Autodesk Fusion 360 part; units mm, degrees
(part 2 of 14)
sketch "Sketch8" plane through (0, 0, 5) normal (0, 0, 1) x (-1, 0, 0)
  spline S0 degree 5 poles (-28.167, 1.1579) (-28.1751, 1.1579) (-28.1914, 1.1578) (-28.2159, 1.1575) (-28.2485, 1.1567) (-28.2892, 1.1551) (-28.33, 1.1529) (-28.3707, 1.1501) (-28.4115, 1.1467) (-28.4523, 1.1427) (-28.493, 1.1383) (-28.5338, 1.1335) (-28.5746, 1.1284) (-28.6154, 1.1228) (-28.6561, 1.117) (-28.6969, 1.1109) (-28.7376, 1.1045) (-28.7783, 1.0977) (-28.8191, 1.0907) (-28.8598, 1.0834) (-28.9005, 1.0758) (-28.9412, 1.0679) (-28.9819, 1.0597) (-29.0226, 1.0513) (-29.0633, 1.0427) (-29.104, 1.0338) (-29.1446, 1.0247) (-29.1853, 1.0153) (-29.2259, 1.0057) (-29.2665, 0.9959) (-29.3071, 0.9858) (-29.3477, 0.9755) (-29.3883, 0.965) (-29.4289, 0.9543) (-29.4694, 0.9434) (-29.5099, 0.9323) (-29.5505, 0.921) (-29.591, 0.9094) (-29.6315, 0.8977) (-29.672, 0.8858) (-29.7124, 0.8737) (-29.7529, 0.8614) (-29.7933, 0.8488) (-29.8337, 0.8361) (-29.8741, 0.8233) (-29.9145, 0.8102) (-29.9549, 0.7969) (-29.9952, 0.7835) (-30.0355, 0.7699) (-30.0759, 0.7561) (-30.1161, 0.7421) (-30.1564, 0.728) (-30.1967, 0.7137) (-30.2369, 0.6992) (-30.2771, 0.6845) (-30.3173, 0.6697) (-30.3575, 0.6547) (-30.3977, 0.6396) (-30.4378, 0.6242) (-30.4779, 0.6087) (-30.518, 0.5931) (-30.5581, 0.5773) (-30.5982, 0.5613) (-30.6382, 0.5451) (-30.6782, 0.5288) (-30.7182, 0.5124) (-30.7582, 0.4958) (-30.7981, 0.479) (-30.838, 0.4621) (-30.8779, 0.445) (-30.9178, 0.4278) (-30.9497, 0.4139) (-30.9736, 0.4034) (-30.9895, 0.3963) (-30.9975, 0.3928) knots 0 0 0 0 0 0 0.01428571 0.02857143 0.04285714 0.05714286 0.07142857 0.08571429 0.1 0.11428571 0.12857143 0.14285714 0.15714286 0.17142857 0.18571429 0.2 0.21428571 0.22857143 0.24285714 0.25714286 0.27142857 0.28571429 0.3 0.31428571 0.32857143 0.34285714 0.35714286 0.37142857 0.38571429 0.4 0.41428571 0.42857143 0.44285714 0.45714286 0.47142857 0.48571429 0.5 0.51428571 0.52857143 0.54285714 0.55714286 0.57142857 0.58571429 0.6 0.61428571 0.62857143 0.64285714 0.65714286 0.67142857 0.68571429 0.7 0.71428571 0.72857143 0.74285714 0.75714286 0.77142857 0.78571429 0.8 0.81428571 0.82857143 0.84285714 0.85714286 0.87142857 0.88571429 0.9 0.91428571 0.92857143 0.94285714 0.95714286 0.97142857 0.98571429 1 1 1 1 1 1
  arc A0 (-30.9975, 0.3928) -> (-30.9975, -0.3928) centre (0, 0) ccw
  spline S1 degree 5 poles (-30.9975, -0.3928) (-30.9895, -0.3963) (-30.9736, -0.4034) (-30.9497, -0.4139) (-30.9178, -0.4278) (-30.8779, -0.445) (-30.838, -0.4621) (-30.7981, -0.479) (-30.7582, -0.4958) (-30.7182, -0.5124) (-30.6782, -0.5288) (-30.6382, -0.5451) (-30.5982, -0.5613) (-30.5581, -0.5773) (-30.518, -0.5931) (-30.4779, -0.6087) (-30.4378, -0.6242) (-30.3977, -0.6396) (-30.3575, -0.6547) (-30.3173, -0.6697) (-30.2771, -0.6845) (-30.2369, -0.6992) (-30.1967, -0.7137) (-30.1564, -0.728) (-30.1161, -0.7421) (-30.0759, -0.7561) (-30.0355, -0.7699) (-29.9952, -0.7835) (-29.9549, -0.7969) (-29.9145, -0.8102) (-29.8741, -0.8233) (-29.8337, -0.8361) (-29.7933, -0.8488) (-29.7529, -0.8614) (-29.7124, -0.8737) (-29.672, -0.8858) (-29.6315, -0.8977) (-29.591, -0.9094) (-29.5505, -0.921) (-29.5099, -0.9323) (-29.4694, -0.9434) (-29.4289, -0.9543) (-29.3883, -0.965) (-29.3477, -0.9755) (-29.3071, -0.9858) (-29.2665, -0.9959) (-29.2259, -1.0057) (-29.1853, -1.0153) (-29.1446, -1.0247) (-29.104, -1.0338) (-29.0633, -1.0427) (-29.0226, -1.0513) (-28.9819, -1.0597) (-28.9412, -1.0679) (-28.9005, -1.0758) (-28.8598, -1.0834) (-28.8191, -1.0907) (-28.7783, -1.0977) (-28.7376, -1.1045) (-28.6969, -1.1109) (-28.6561, -1.117) (-28.6154, -1.1228) (-28.5746, -1.1284) (-28.5338, -1.1335) (-28.493, -1.1383) (-28.4523, -1.1427) (-28.4115, -1.1467) (-28.3707, -1.1501) (-28.33, -1.1529) (-28.2892, -1.1551) (-28.2485, -1.1567) (-28.2159, -1.1575) (-28.1914, -1.1578) (-28.1751, -1.1579) (-28.167, -1.1579) knots -1 -1 -1 -1 -1 -1 -0.98571429 -0.97142857 -0.95714286 -0.94285714 -0.92857143 -0.91428571 -0.9 -0.88571429 -0.87142857 -0.85714286 -0.84285714 -0.82857143 -0.81428571 -0.8 -0.78571429 -0.77142857 -0.75714286 -0.74285714 -0.72857143 -0.71428571 -0.7 -0.68571429 -0.67142857 -0.65714286 -0.64285714 -0.62857143 -0.61428571 -0.6 -0.58571429 -0.57142857 -0.55714286 -0.54285714 -0.52857143 -0.51428571 -0.5 -0.48571429 -0.47142857 -0.45714286 -0.44285714 -0.42857143 -0.41428571 -0.4 -0.38571429 -0.37142857 -0.35714286 -0.34285714 -0.32857143 -0.31428571 -0.3 -0.28571429 -0.27142857 -0.25714286 -0.24285714 -0.22857143 -0.21428571 -0.2 -0.18571429 -0.17142857 -0.15714286 -0.14285714 -0.12857143 -0.11428571 -0.1 -0.08571429 -0.07142857 -0.05714286 -0.04285714 -0.02857143 -0.01428571 0 0 0 0 0 0
  spline S2 degree 5 poles (-28.1337, -1.7927) (-28.1418, -1.7936) (-28.158, -1.7954) (-28.1823, -1.7982) (-28.2146, -1.8024) (-28.255, -1.8083) (-28.2953, -1.8147) (-28.3355, -1.8218) (-28.3757, -1.8294) (-28.4159, -1.8376) (-28.4559, -1.8462) (-28.496, -1.8553) (-28.536, -1.8647) (-28.576, -1.8744) (-28.6159, -1.8845) (-28.6558, -1.8948) (-28.6956, -1.9055) (-28.7354, -1.9164) (-28.7752, -1.9277) (-28.815, -1.9392) (-28.8546, -1.9511) (-28.8943, -1.9632) (-28.9339, -1.9755) (-28.9735, -1.9881) (-29.0131, -2.001) (-29.0526, -2.0141) (-29.0921, -2.0274) (-29.1315, -2.041) (-29.1709, -2.0548) (-29.2103, -2.0688) (-29.2496, -2.083) (-29.2889, -2.0975) (-29.3282, -2.1122) (-29.3674, -2.127) (-29.4066, -2.1421) (-29.4457, -2.1574) (-29.4849, -2.1729) (-29.5239, -2.1886) (-29.563, -2.2045) (-29.602, -2.2206) (-29.641, -2.2369) (-29.6799, -2.2534) (-29.7188, -2.2701) (-29.7577, -2.2869) (-29.7965, -2.3039) (-29.8353, -2.3212) (-29.8741, -2.3386) (-29.9128, -2.3561) (-29.9515, -2.3739) (-29.9901, -2.3918) (-30.0287, -2.4099) (-30.0673, -2.4282) (-30.1059, -2.4466) (-30.1444, -2.4653) (-30.1828, -2.484) (-30.2213, -2.503) (-30.2596, -2.5221) (-30.298, -2.5414) (-30.3363, -2.5608) (-30.3746, -2.5804) (-30.4128, -2.6002) (-30.451, -2.6201) (-30.4892, -2.6402) (-30.5273, -2.6604) (-30.5654, -2.6808) (-30.6035, -2.7013) (-30.6415, -2.722) (-30.6795, -2.7429) (-30.7174, -2.7639) (-30.7553, -2.7851) (-30.7932, -2.8064) (-30.8234, -2.8235) (-30.8461, -2.8365) (-30.8612, -2.8451) (-30.8688, -2.8495) knots 0 0 0 0 0 0 0.01428571 0.02857143 0.04285714 0.05714286 0.07142857 0.08571429 0.1 0.11428571 0.12857143 0.14285714 0.15714286 0.17142857 0.18571429 0.2 0.21428571 0.22857143 0.24285714 0.25714286 0.27142857 0.28571429 0.3 0.31428571 0.32857143 0.34285714 0.35714286 0.37142857 0.38571429 0.4 0.41428571 0.42857143 0.44285714 0.45714286 0.47142857 0.48571429 0.5 0.51428571 0.52857143 0.54285714 0.55714286 0.57142857 0.58571429 0.6 0.61428571 0.62857143 0.64285714 0.65714286 0.67142857 0.68571429 0.7 0.71428571 0.72857143 0.74285714 0.75714286 0.77142857 0.78571429 0.8 0.81428571 0.82857143 0.84285714 0.85714286 0.87142857 0.88571429 0.9 0.91428571 0.92857143 0.94285714 0.95714286 0.97142857 0.98571429 1 1 1 1 1 1
  arc A1 (-30.8688, -2.8495) -> (-30.7866, -3.6308) centre (0, 0) ccw
  spline S3 degree 5 poles (-30.7866, -3.6308) (-30.7784, -3.6335) (-30.7618, -3.6388) (-30.7369, -3.6467) (-30.7037, -3.6572) (-30.6623, -3.6702) (-30.6208, -3.683) (-30.5793, -3.6957) (-30.5379, -3.7082) (-30.4964, -3.7205) (-30.4549, -3.7327) (-30.4134, -3.7447) (-30.3719, -3.7566) (-30.3304, -3.7683) (-30.2889, -3.7798) (-30.2473, -3.7912) (-30.2058, -3.8024) (-30.1643, -3.8135) (-30.1228, -3.8244) (-30.0812, -3.8351) (-30.0397, -3.8456) (-29.9982, -3.856) (-29.9567, -3.8662) (-29.9151, -3.8762) (-29.8736, -3.8861) (-29.8321, -3.8958) (-29.7905, -3.9053) (-29.749, -3.9146) (-29.7075, -3.9237) (-29.6659, -3.9327) (-29.6244, -3.9415) (-29.5829, -3.95) (-29.5414, -3.9584) (-29.4998, -3.9667) (-29.4583, -3.9747) (-29.4168, -3.9825) (-29.3753, -3.9901) (-29.3338, -3.9976) (-29.2923, -4.0048) (-29.2508, -4.0118) (-29.2094, -4.0186) (-29.1679, -4.0253) (-29.1264, -4.0317) (-29.085, -4.0379) (-29.0435, -4.0438) (-29.0021, -4.0496) (-28.9607, -4.0551) (-28.9192, -4.0604) (-28.8778, -4.0655) (-28.8365, -4.0703) (-28.7951, -4.0749) (-28.7537, -4.0792) (-28.7124, -4.0833) (-28.6711, -4.0872) (-28.6298, -4.0908) (-28.5885, -4.0941) (-28.5472, -4.0971) (-28.506, -4.0999) (-28.4647, -4.1023) (-28.4235, -4.1044) (-28.3824, -4.1063) (-28.3412, -4.1078) (-28.3001, -4.109) (-28.259, -4.1099) (-28.218, -4.1104) (-28.177, -4.1106) (-28.136, -4.1102) (-28.0951, -4.1093) (-28.0543, -4.1078) (-28.0135, -4.1058) (-27.9728, -4.1031) (-27.9403, -4.1005) (-27.916, -4.0983) (-27.8998, -4.0966) (-27.8917, -4.0958) knots -1 -1 -1 -1 -1 -1 -0.98571429 -0.97142857 -0.95714286 -0.94285714 -0.92857143 -0.91428571 -0.9 -0.88571429 -0.87142857 -0.85714286 -0.84285714 -0.82857143 -0.81428571 -0.8 -0.78571429 -0.77142857 -0.75714286 -0.74285714 -0.72857143 -0.71428571 -0.7 -0.68571429 -0.67142857 -0.65714286 -0.64285714 -0.62857143 -0.61428571 -0.6 -0.58571429 -0.57142857 -0.55714286 -0.54285714 -0.52857143 -0.51428571 -0.5 -0.48571429 -0.47142857 -0.45714286 -0.44285714 -0.42857143 -0.41428571 -0.4 -0.38571429 -0.37142857 -0.35714286 -0.34285714 -0.32857143 -0.31428571 -0.3 -0.28571429 -0.27142857 -0.25714286 -0.24285714 -0.22857143 -0.21428571 -0.2 -0.18571429 -0.17142857 -0.15714286 -0.14285714 -0.12857143 -0.11428571 -0.1 -0.08571429 -0.07142857 -0.05714286 -0.04285714 -0.02857143 -0.01428571 0 0 0 0 0 0
  spline S4 degree 5 poles (-27.7922, -4.7237) (-27.8002, -4.7254) (-27.8161, -4.7288) (-27.8399, -4.7342) (-27.8717, -4.7418) (-27.9112, -4.7518) (-27.9506, -4.7625) (-27.9899, -4.7737) (-28.029, -4.7855) (-28.0681, -4.7978) (-28.1071, -4.8106) (-28.146, -4.8237) (-28.1848, -4.8373) (-28.2235, -4.8512) (-28.2621, -4.8653) (-28.3007, -4.8798) (-28.3393, -4.8946) (-28.3777, -4.9096) (-28.4161, -4.925) (-28.4544, -4.9406) (-28.4926, -4.9565) (-28.5308, -4.9727) (-28.5689, -4.9891) (-28.607, -5.0058) (-28.645, -5.0227) (-28.6829, -5.0399) (-28.7208, -5.0572) (-28.7586, -5.0749) (-28.7963, -5.0927) (-28.834, -5.1107) (-28.8716, -5.129) (-28.9092, -5.1475) (-28.9467, -5.1662) (-28.9842, -5.1851) (-29.0216, -5.2042) (-29.0589, -5.2235) (-29.0962, -5.243) (-29.1334, -5.2627) (-29.1706, -5.2826) (-29.2077, -5.3027) (-29.2448, -5.323) (-29.2818, -5.3434) (-29.3187, -5.3641) (-29.3556, -5.3849) (-29.3925, -5.4059) (-29.4292, -5.4271) (-29.466, -5.4484) (-29.5026, -5.47) (-29.5393, -5.4917) (-29.5758, -5.5135) (-29.6123, -5.5356) (-29.6488, -5.5578) (-29.6852, -5.5802) (-29.7215, -5.6027) (-29.7578, -5.6254) (-29.7941, -5.6483) (-29.8303, -5.6713) (-29.8664, -5.6945) (-29.9025, -5.7178) (-29.9385, -5.7413) (-29.9744, -5.7649) (-30.0104, -5.7887) (-30.0462, -5.8127) (-30.082, -5.8368) (-30.1178, -5.8611) (-30.1535, -5.8855) (-30.1891, -5.91) (-30.2247, -5.9348) (-30.2602, -5.9596) (-30.2957, -5.9846) (-30.3311, -6.0097) (-30.3594, -6.03) (-30.3806, -6.0452) (-30.3948, -6.0554) (-30.4018, -6.0605) knots 0 0 0 0 0 0 0.01428571 0.02857143 0.04285714 0.05714286 0.07142857 0.08571429 0.1 0.11428571 0.12857143 0.14285714 0.15714286 0.17142857 0.18571429 0.2 0.21428571 0.22857143 0.24285714 0.25714286 0.27142857 0.28571429 0.3 0.31428571 0.32857143 0.34285714 0.35714286 0.37142857 0.38571429 0.4 0.41428571 0.42857143 0.44285714 0.45714286 0.47142857 0.48571429 0.5 0.51428571 0.52857143 0.54285714 0.55714286 0.57142857 0.58571429 0.6 0.61428571 0.62857143 0.64285714 0.65714286 0.67142857 0.68571429 0.7 0.71428571 0.72857143 0.74285714 0.75714286 0.77142857 0.78571429 0.8 0.81428571 0.82857143 0.84285714 0.85714286 0.87142857 0.88571429 0.9 0.91428571 0.92857143 0.94285714 0.95714286 0.97142857 0.98571429 1 1 1 1 1 1
  arc A2 (-30.4018, -6.0605) -> (-30.2385, -6.829) centre (0, 0) ccw
  spline S5 degree 5 poles (-30.2385, -6.829) (-30.2299, -6.8308) (-30.2129, -6.8343) (-30.1873, -6.8396) (-30.1533, -6.8466) (-30.1107, -6.8552) (-30.0681, -6.8636) (-30.0255, -6.8718) (-29.983, -6.8799) (-29.9404, -6.8879) (-29.8979, -6.8956) (-29.8553, -6.9033) (-29.8128, -6.9107) (-29.7703, -6.918) (-29.7278, -6.9252) (-29.6854, -6.9321) (-29.6429, -6.939) (-29.6004, -6.9456) (-29.558, -6.9521) (-29.5156, -6.9584) (-29.4732, -6.9646) (-29.4308, -6.9705) (-29.3884, -6.9763) (-29.3461, -6.982) (-29.3037, -6.9874) (-29.2614, -6.9927) (-29.2191, -6.9978) (-29.1768, -7.0027) (-29.1346, -7.0075) (-29.0923, -7.0121) (-29.0501, -7.0165) (-29.0079, -7.0207) (-28.9658, -7.0247) (-28.9236, -7.0285) (-28.8815, -7.0321) (-28.8394, -7.0356) (-28.7973, -7.0388) (-28.7553, -7.0419) (-28.7132, -7.0447) (-28.6712, -7.0474) (-28.6293, -7.0498) (-28.5873, -7.0521) (-28.5454, -7.0541) (-28.5036, -7.0559) (-28.4617, -7.0576) (-28.4199, -7.059) (-28.3781, -7.0601) (-28.3364, -7.0611) (-28.2947, -7.0618) (-28.253, -7.0622) (-28.2114, -7.0625) (-28.1698, -7.0625) (-28.1283, -7.0622) (-28.0868, -7.0618) (-28.0453, -7.061) (-28.0039, -7.06) (-27.9625, -7.0587) (-27.9212, -7.0571) (-27.88, -7.0552) (-27.8388, -7.053) (-27.7977, -7.0505) (-27.7566, -7.0478) (-27.7156, -7.0447) (-27.6746, -7.0413) (-27.6337, -7.0375) (-27.5929, -7.0333) (-27.5522, -7.0287) (-27.5117, -7.0235) (-27.4712, -7.0178) (-27.4309, -7.0115) (-27.3907, -7.0046) (-27.3586, -6.9986) (-27.3347, -6.9938) (-27.3187, -6.9905) (-27.3107, -6.9888) knots -1 -1 -1 -1 -1 -1 -0.98571429 -0.97142857 -0.95714286 -0.94285714 -0.92857143 -0.91428571 -0.9 -0.88571429 -0.87142857 -0.85714286 -0.84285714 -0.82857143 -0.81428571 -0.8 -0.78571429 -0.77142857 -0.75714286 -0.74285714 -0.72857143 -0.71428571 -0.7 -0.68571429 -0.67142857 -0.65714286 -0.64285714 -0.62857143 -0.61428571 -0.6 -0.58571429 -0.57142857 -0.55714286 -0.54285714 -0.52857143 -0.51428571 -0.5 -0.48571429 -0.47142857 -0.45714286 -0.44285714 -0.42857143 -0.41428571 -0.4 -0.38571429 -0.37142857 -0.35714286 -0.34285714 -0.32857143 -0.31428571 -0.3 -0.28571429 -0.27142857 -0.25714286 -0.24285714 -0.22857143 -0.21428571 -0.2 -0.18571429 -0.17142857 -0.15714286 -0.14285714 -0.12857143 -0.11428571 -0.1 -0.08571429 -0.07142857 -0.05714286 -0.04285714 -0.02857143 -0.01428571 0 0 0 0 0 0
  spline S6 degree 5 poles (-27.1462, -7.6029) (-27.1539, -7.6054) (-27.1694, -7.6105) (-27.1926, -7.6184) (-27.2233, -7.6292) (-27.2616, -7.6433) (-27.2997, -7.658) (-27.3376, -7.6733) (-27.3753, -7.6891) (-27.4128, -7.7054) (-27.4503, -7.7222) (-27.4876, -7.7394) (-27.5247, -7.7569) (-27.5618, -7.7747) (-27.5988, -7.7929) (-27.6356, -7.8113) (-27.6724, -7.83) (-27.7091, -7.849) (-27.7456, -7.8683) (-27.7821, -7.8878) (-27.8185, -7.9076) (-27.8547, -7.9277) (-27.8909, -7.9481) (-27.927, -7.9686) (-27.963, -7.9894) (-27.999, -8.0104) (-28.0348, -8.0317) (-28.0706, -8.0531) (-28.1062, -8.0748) (-28.1418, -8.0967) (-28.1774, -8.1188) (-28.2128, -8.1412) (-28.2481, -8.1637) (-28.2834, -8.1864) (-28.3186, -8.2093) (-28.3537, -8.2324) (-28.3888, -8.2557) (-28.4237, -8.2792) (-28.4586, -8.3028) (-28.4934, -8.3267) (-28.5282, -8.3507) (-28.5628, -8.3749) (-28.5974, -8.3993) (-28.6319, -8.4239) (-28.6664, -8.4486) (-28.7007, -8.4735) (-28.735, -8.4986) (-28.7693, -8.5239) (-28.8034, -8.5493) (-28.8375, -8.5748) (-28.8715, -8.6006) (-28.9054, -8.6265) (-28.9393, -8.6525) (-28.9731, -8.6787) (-29.0068, -8.7051) (-29.0405, -8.7316) (-29.074, -8.7583) (-29.1075, -8.7851) (-29.141, -8.8121) (-29.1743, -8.8393) (-29.2076, -8.8665) (-29.2409, -8.894) (-29.274, -8.9215) (-29.3071, -8.9493) (-29.3401, -8.9771) (-29.3731, -9.0051) (-29.406, -9.0333) (-29.4388, -9.0616) (-29.4715, -9.09) (-29.5042, -9.1186) (-29.5368, -9.1473) (-29.5628, -9.1704) (-29.5823, -9.1877) (-29.5953, -9.1994) (-29.6018, -9.2052) knots 0 0 0 0 0 0 0.01428571 0.02857143 0.04285714 0.05714286 0.07142857 0.08571429 0.1 0.11428571 0.12857143 0.14285714 0.15714286 0.17142857 0.18571429 0.2 0.21428571 0.22857143 0.24285714 0.25714286 0.27142857 0.28571429 0.3 0.31428571 0.32857143 0.34285714 0.35714286 0.37142857 0.38571429 0.4 0.41428571 0.42857143 0.44285714 0.45714286 0.47142857 0.48571429 0.5 0.51428571 0.52857143 0.54285714 0.55714286 0.57142857 0.58571429 0.6 0.61428571 0.62857143 0.64285714 0.65714286 0.67142857 0.68571429 0.7 0.71428571 0.72857143 0.74285714 0.75714286 0.77142857 0.78571429 0.8 0.81428571 0.82857143 0.84285714 0.85714286 0.87142857 0.88571429 0.9 0.91428571 0.92857143 0.94285714 0.95714286 0.97142857 0.98571429 1 1 1 1 1 1
  arc A3 (-29.6018, -9.2052) -> (-29.359, -9.9524) centre (0, 0) ccw
  spline S7 degree 5 poles (-29.359, -9.9524) (-29.3503, -9.9532) (-29.333, -9.955) (-29.307, -9.9576) (-29.2724, -9.961) (-29.2292, -9.965) (-29.1859, -9.9689) (-29.1427, -9.9727) (-29.0996, -9.9763) (-29.0564, -9.9798) (-29.0133, -9.983) (-28.9702, -9.9862) (-28.9271, -9.9892) (-28.8841, -9.992) (-28.8411, -9.9946) (-28.7981, -9.9971) (-28.7552, -9.9995) (-28.7123, -10.0016) (-28.6694, -10.0037) (-28.6265, -10.0055) (-28.5837, -10.0072) (-28.541, -10.0087) (-28.4982, -10.01) (-28.4555, -10.0112) (-28.4128, -10.0122) (-28.3702, -10.0131) (-28.3276, -10.0137) (-28.285, -10.0142) (-28.2425, -10.0145) (-28.2, -10.0146) (-28.1576, -10.0146) (-28.1152, -10.0144) (-28.0728, -10.0139) (-28.0305, -10.0133) (-27.9882, -10.0126) (-27.946, -10.0116) (-27.9038, -10.0104) (-27.8617, -10.0091) (-27.8196, -10.0075) (-27.7775, -10.0057) (-27.7355, -10.0038) (-27.6936, -10.0016) (-27.6517, -9.9993) (-27.6099, -9.9967) (-27.5681, -9.994) (-27.5264, -9.991) (-27.4847, -9.9878) (-27.4431, -9.9843) (-27.4015, -9.9807) (-27.3601, -9.9768) (-27.3186, -9.9727) (-27.2773, -9.9683) (-27.236, -9.9638) (-27.1948, -9.9589) (-27.1536, -9.9539) (-27.1125, -9.9485) (-27.0715, -9.9429) (-27.0306, -9.937) (-26.9898, -9.9308) (-26.9491, -9.9243) (-26.9084, -9.9176) (-26.8678, -9.9105) (-26.8274, -9.9032) (-26.787, -9.8955) (-26.7467, -9.8875) (-26.7066, -9.879) (-26.6666, -9.8702) (-26.6268, -9.8608) (-26.5871, -9.8509) (-26.5477, -9.8404) (-26.5084, -9.8293) (-26.4772, -9.82) (-26.4539, -9.8128) (-26.4383, -9.8078) (-26.4306, -9.8053) knots -1 -1 -1 -1 -1 -1 -0.98571429 -0.97142857 -0.95714286 -0.94285714 -0.92857143 -0.91428571 -0.9 -0.88571429 -0.87142857 -0.85714286 -0.84285714 -0.82857143 -0.81428571 -0.8 -0.78571429 -0.77142857 -0.75714286 -0.74285714 -0.72857143 -0.71428571 -0.7 -0.68571429 -0.67142857 -0.65714286 -0.64285714 -0.62857143 -0.61428571 -0.6 -0.58571429 -0.57142857 -0.55714286 -0.54285714 -0.52857143 -0.51428571 -0.5 -0.48571429 -0.47142857 -0.45714286 -0.44285714 -0.42857143 -0.41428571 -0.4 -0.38571429 -0.37142857 -0.35714286 -0.34285714 -0.32857143 -0.31428571 -0.3 -0.28571429 -0.27142857 -0.25714286 -0.24285714 -0.22857143 -0.21428571 -0.2 -0.18571429 -0.17142857 -0.15714286 -0.14285714 -0.12857143 -0.11428571 -0.1 -0.08571429 -0.07142857 -0.05714286 -0.04285714 -0.02857143 -0.01428571 0 0 0 0 0 0
  spline S8 degree 5 poles (-26.2028, -10.3988) (-26.2102, -10.4021) (-26.2251, -10.4088) (-26.2473, -10.419) (-26.2767, -10.433) (-26.3133, -10.451) (-26.3496, -10.4696) (-26.3857, -10.4888) (-26.4216, -10.5085) (-26.4572, -10.5286) (-26.4927, -10.5492) (-26.528, -10.5702) (-26.5631, -10.5915) (-26.5981, -10.6131) (-26.633, -10.635) (-26.6677, -10.6572) (-26.7023, -10.6797) (-26.7368, -10.7024) (-26.7712, -10.7254) (-26.8054, -10.7486) (-26.8395, -10.7721) (-26.8735, -10.7959) (-26.9073, -10.8199) (-26.9411, -10.8441) (-26.9747, -10.8686) (-27.0083, -10.8932) (-27.0417, -10.9181) (-27.075, -10.9432) (-27.1082, -10.9685) (-27.1413, -10.994) (-27.1743, -11.0197) (-27.2073, -11.0456) (-27.2401, -11.0717) (-27.2728, -11.098) (-27.3054, -11.1244) (-27.3379, -11.1511) (-27.3703, -11.1779) (-27.4026, -11.2049) (-27.4348, -11.2321) (-27.467, -11.2595) (-27.499, -11.287) (-27.5309, -11.3147) (-27.5628, -11.3426) (-27.5946, -11.3706) (-27.6262, -11.3988) (-27.6578, -11.4272) (-27.6893, -11.4557) (-27.7207, -11.4844) (-27.752, -11.5132) (-27.7832, -11.5422) (-27.8143, -11.5714) (-27.8454, -11.6007) (-27.8763, -11.6301) (-27.9072, -11.6597) (-27.938, -11.6895) (-27.9687, -11.7194) (-27.9993, -11.7494) (-28.0298, -11.7796) (-28.0602, -11.8099) (-28.0906, -11.8404) (-28.1208, -11.871) (-28.151, -11.9018) (-28.1811, -11.9326) (-28.2111, -11.9637) (-28.241, -11.9948) (-28.2709, -12.0261) (-28.3006, -12.0576) (-28.3303, -12.0891) (-28.3599, -12.1208) (-28.3894, -12.1527) (-28.4188, -12.1846) (-28.4423, -12.2103) (-28.4599, -12.2296) (-28.4716, -12.2425) (-28.4774, -12.249) knots 0 0 0 0 0 0 0.01428571 0.02857143 0.04285714 0.05714286 0.07142857 0.08571429 0.1 0.11428571 0.12857143 0.14285714 0.15714286 0.17142857 0.18571429 0.2 0.21428571 0.22857143 0.24285714 0.25714286 0.27142857 0.28571429 0.3 0.31428571 0.32857143 0.34285714 0.35714286 0.37142857 0.38571429 0.4 0.41428571 0.42857143 0.44285714 0.45714286 0.47142857 0.48571429 0.5 0.51428571 0.52857143 0.54285714 0.55714286 0.57142857 0.58571429 0.6 0.61428571 0.62857143 0.64285714 0.65714286 0.67142857 0.68571429 0.7 0.71428571 0.72857143 0.74285714 0.75714286 0.77142857 0.78571429 0.8 0.81428571 0.82857143 0.84285714 0.85714286 0.87142857 0.88571429 0.9 0.91428571 0.92857143 0.94285714 0.95714286 0.97142857 0.98571429 1 1 1 1 1 1
  arc A4 (-28.4774, -12.249) -> (-28.1579, -12.9667) centre (0, 0) ccw
  spline S9 degree 5 poles (-28.1579, -12.9667) (-28.1492, -12.9667) (-28.1317, -12.9666) (-28.1056, -12.9665) (-28.0708, -12.9662) (-28.0274, -12.9657) (-27.984, -12.9651) (-27.9407, -12.9643) (-27.8973, -12.9634) (-27.8541, -12.9623) (-27.8108, -12.9611) (-27.7677, -12.9597) (-27.7245, -12.9581) (-27.6814, -12.9565) (-27.6384, -12.9546) (-27.5954, -12.9526) (-27.5524, -12.9504) (-27.5095, -12.9481) (-27.4667, -12.9456) (-27.4239, -12.943) (-27.3811, -12.9402) (-27.3384, -12.9372) (-27.2958, -12.9341) (-27.2532, -12.9308) (-27.2106, -12.9273) (-27.1681, -12.9237) (-27.1257, -12.9199) (-27.0833, -12.9159) (-27.041, -12.9118) (-26.9987, -12.9075) (-26.9565, -12.903) (-26.9144, -12.8983) (-26.8723, -12.8935) (-26.8303, -12.8885) (-26.7883, -12.8833) (-26.7464, -12.8779) (-26.7046, -12.8723) (-26.6628, -12.8666) (-26.6211, -12.8606) (-26.5795, -12.8545) (-26.5379, -12.8482) (-26.4964, -12.8416) (-26.455, -12.8349) (-26.4137, -12.828) (-26.3724, -12.8209) (-26.3312, -12.8135) (-26.2901, -12.806) (-26.2491, -12.7982) (-26.2082, -12.7902) (-26.1673, -12.7821) (-26.1265, -12.7736) (-26.0859, -12.765) (-26.0453, -12.7561) (-26.0048, -12.747) (-25.9644, -12.7377) (-25.9241, -12.728) (-25.8839, -12.7182) (-25.8438, -12.708) (-25.8039, -12.6976) (-25.7641, -12.6869) (-25.7243, -12.6759) (-25.6847, -12.6647) (-25.6452, -12.6531) (-25.6059, -12.6413) (-25.5667, -12.6291) (-25.5277, -12.6165) (-25.4888, -12.6035) (-25.4502, -12.59) (-25.4118, -12.576) (-25.3737, -12.5615) (-25.3358, -12.5464) (-25.3057, -12.5338) (-25.2832, -12.5242) (-25.2683, -12.5176) (-25.2609, -12.5143) knots -1 -1 -1 -1 -1 -1 -0.98571429 -0.97142857 -0.95714286 -0.94285714 -0.92857143 -0.91428571 -0.9 -0.88571429 -0.87142857 -0.85714286 -0.84285714 -0.82857143 -0.81428571 -0.8 -0.78571429 -0.77142857 -0.75714286 -0.74285714 -0.72857143 -0.71428571 -0.7 -0.68571429 -0.67142857 -0.65714286 -0.64285714 -0.62857143 -0.61428571 -0.6 -0.58571429 -0.57142857 -0.55714286 -0.54285714 -0.52857143 -0.51428571 -0.5 -0.48571429 -0.47142857 -0.45714286 -0.44285714 -0.42857143 -0.41428571 -0.4 -0.38571429 -0.37142857 -0.35714286 -0.34285714 -0.32857143 -0.31428571 -0.3 -0.28571429 -0.27142857 -0.25714286 -0.24285714 -0.22857143 -0.21428571 -0.2 -0.18571429 -0.17142857 -0.15714286 -0.14285714 -0.12857143 -0.11428571 -0.1 -0.08571429 -0.07142857 -0.05714286 -0.04285714 -0.02857143 -0.01428571 0 0 0 0 0 0
  spline S10 degree 5 poles (-24.9723, -13.0807) (-24.9793, -13.0848) (-24.9934, -13.093) (-25.0144, -13.1055) (-25.0422, -13.1225) (-25.0767, -13.1443) (-25.1109, -13.1666) (-25.1448, -13.1894) (-25.1784, -13.2127) (-25.2118, -13.2365) (-25.2449, -13.2607) (-25.2778, -13.2852) (-25.3105, -13.3101) (-25.343, -13.3353) (-25.3754, -13.3607) (-25.4077, -13.3864) (-25.4397, -13.4123) (-25.4716, -13.4385) (-25.5034, -13.465) (-25.535, -13.4917) (-25.5665, -13.5186) (-25.5978, -13.5458) (-25.6289, -13.5732) (-25.66, -13.6008) (-25.6909, -13.6287) (-25.7217, -13.6567) (-25.7523, -13.6849) (-25.7828, -13.7134) (-25.8132, -13.742) (-25.8435, -13.7708) (-25.8736, -13.7998) (-25.9036, -13.829) (-25.9335, -13.8584) (-25.9633, -13.8879) (-25.993, -13.9177) (-26.0225, -13.9476) (-26.0519, -13.9776) (-26.0813, -14.0079) (-26.1105, -14.0383) (-26.1396, -14.0689) (-26.1685, -14.0996) (-26.1974, -14.1305) (-26.2262, -14.1615) (-26.2548, -14.1927) (-26.2834, -14.2241) (-26.3118, -14.2556) (-26.3401, -14.2873) (-26.3684, -14.3191) (-26.3965, -14.351) (-26.4245, -14.3831) (-26.4524, -14.4154) (-26.4802, -14.4477) (-26.5079, -14.4803) (-26.5355, -14.5129) (-26.563, -14.5457) (-26.5904, -14.5787) (-26.6177, -14.6118) (-26.6449, -14.645) (-26.672, -14.6783) (-26.699, -14.7118) (-26.7259, -14.7454) (-26.7527, -14.7791) (-26.7794, -14.813) (-26.806, -14.847) (-26.8325, -14.8811) (-26.8589, -14.9154) (-26.8852, -14.9497) (-26.9115, -14.9842) (-26.9376, -15.0188) (-26.9636, -15.0536) (-26.9895, -15.0884) (-27.0102, -15.1164) (-27.0256, -15.1375) (-27.0359, -15.1515) (-27.041, -15.1586) knots 0 0 0 0 0 0 0.01428571 0.02857143 0.04285714 0.05714286 0.07142857 0.08571429 0.1 0.11428571 0.12857143 0.14285714 0.15714286 0.17142857 0.18571429 0.2 0.21428571 0.22857143 0.24285714 0.25714286 0.27142857 0.28571429 0.3 0.31428571 0.32857143 0.34285714 0.35714286 0.37142857 0.38571429 0.4 0.41428571 0.42857143 0.44285714 0.45714286 0.47142857 0.48571429 0.5 0.51428571 0.52857143 0.54285714 0.55714286 0.57142857 0.58571429 0.6 0.61428571 0.62857143 0.64285714 0.65714286 0.67142857 0.68571429 0.7 0.71428571 0.72857143 0.74285714 0.75714286 0.77142857 0.78571429 0.8 0.81428571 0.82857143 0.84285714 0.85714286 0.87142857 0.88571429 0.9 0.91428571 0.92857143 0.94285714 0.95714286 0.97142857 0.98571429 1 1 1 1 1 1
  arc A5 (-27.041, -15.1586) -> (-26.6482, -15.8389) centre (0, 0) ccw
  spline S11 degree 5 poles (-26.6482, -15.8389) (-26.6396, -15.838) (-26.6223, -15.8361) (-26.5963, -15.8333) (-26.5617, -15.8294) (-26.5186, -15.8244) (-26.4755, -15.8192) (-26.4325, -15.8139) (-26.3895, -15.8084) (-26.3466, -15.8028) (-26.3037, -15.7971) (-26.2609, -15.7912) (-26.2181, -15.7852) (-26.1755, -15.779) (-26.1329, -15.7726) (-26.0903, -15.7661) (-26.0478, -15.7595) (-26.0054, -15.7527) (-25.963, -15.7458) (-25.9207, -15.7387) (-25.8785, -15.7314) (-25.8363, -15.724) (-25.7942, -15.7164) (-25.7522, -15.7087) (-25.7103, -15.7008) (-25.6684, -15.6927) (-25.6266, -15.6845) (-25.5849, -15.6762) (-25.5432, -15.6676) (-25.5016, -15.6589) (-25.4601, -15.65) (-25.4187, -15.641) (-25.3773, -15.6318) (-25.3361, -15.6224) (-25.2949, -15.6128) (-25.2538, -15.6031) (-25.2128, -15.5932) (-25.1718, -15.5831) (-25.131, -15.5728) (-25.0902, -15.5624) (-25.0495, -15.5517) (-25.009, -15.5409) (-24.9685, -15.5299) (-24.9281, -15.5187) (-24.8878, -15.5073) (-24.8476, -15.4957) (-24.8075, -15.4839) (-24.7675, -15.4719) (-24.7276, -15.4597) (-24.6879, -15.4473) (-24.6482, -15.4346) (-24.6087, -15.4218) (-24.5692, -15.4087) (-24.5299, -15.3954) (-24.4907, -15.3819) (-24.4516, -15.3681) (-24.4127, -15.3541) (-24.3739, -15.3398) (-24.3353, -15.3253) (-24.2968, -15.3105) (-24.2584, -15.2954) (-24.2202, -15.2801) (-24.1821, -15.2645) (-24.1442, -15.2486) (-24.1065, -15.2324) (-24.069, -15.2158) (-24.0318, -15.1988) (-23.9948, -15.1813) (-23.958, -15.1634) (-23.9216, -15.1449) (-23.8855, -15.126) (-23.8569, -15.1103) (-23.8356, -15.0984) (-23.8215, -15.0903) (-23.8144, -15.0862) knots -1 -1 -1 -1 -1 -1 -0.98571429 -0.97142857 -0.95714286 -0.94285714 -0.92857143 -0.91428571 -0.9 -0.88571429 -0.87142857 -0.85714286 -0.84285714 -0.82857143 -0.81428571 -0.8 -0.78571429 -0.77142857 -0.75714286 -0.74285714 -0.72857143 -0.71428571 -0.7 -0.68571429 -0.67142857 -0.65714286 -0.64285714 -0.62857143 -0.61428571 -0.6 -0.58571429 -0.57142857 -0.55714286 -0.54285714 -0.52857143 -0.51428571 -0.5 -0.48571429 -0.47142857 -0.45714286 -0.44285714 -0.42857143 -0.41428571 -0.4 -0.38571429 -0.37142857 -0.35714286 -0.34285714 -0.32857143 -0.31428571 -0.3 -0.28571429 -0.27142857 -0.25714286 -0.24285714 -0.22857143 -0.21428571 -0.2 -0.18571429 -0.17142857 -0.15714286 -0.14285714 -0.12857143 -0.11428571 -0.1 -0.08571429 -0.07142857 -0.05714286 -0.04285714 -0.02857143 -0.01428571 0 0 0 0 0 0
  spline S12 degree 5 poles (-23.4682, -15.6194) (-23.4747, -15.6242) (-23.4879, -15.6338) (-23.5075, -15.6485) (-23.5334, -15.6682) (-23.5654, -15.6935) (-23.5971, -15.7192) (-23.6284, -15.7455) (-23.6594, -15.7722) (-23.6901, -15.7993) (-23.7205, -15.8269) (-23.7506, -15.8547) (-23.7806, -15.8829) (-23.8103, -15.9113) (-23.8398, -15.94) (-23.8692, -15.9689) (-23.8984, -15.998) (-23.9274, -16.0274) (-23.9562, -16.057) (-23.9849, -16.0869) (-24.0133, -16.117) (-24.0416, -16.1473) (-24.0698, -16.1778) (-24.0977, -16.2085) (-24.1256, -16.2394) (-24.1532, -16.2705) (-24.1808, -16.3018) (-24.2081, -16.3333) (-24.2354, -16.3649) (-24.2625, -16.3967) (-24.2894, -16.4288) (-24.3162, -16.4609) (-24.3429, -16.4933) (-24.3694, -16.5258) (-24.3958, -16.5584) (-24.422, -16.5913) (-24.4482, -16.6242) (-24.4742, -16.6574) (-24.5, -16.6907) (-24.5258, -16.7241) (-24.5514, -16.7577) (-24.5769, -16.7915) (-24.6022, -16.8253) (-24.6275, -16.8594) (-24.6526, -16.8935) (-24.6776, -16.9278) (-24.7024, -16.9623) (-24.7272, -16.9969) (-24.7518, -17.0316) (-24.7763, -17.0664) (-24.8007, -17.1014) (-24.825, -17.1365) (-24.8491, -17.1718) (-24.8732, -17.2072) (-24.8971, -17.2426) (-24.9209, -17.2783) (-24.9446, -17.314) (-24.9682, -17.3499) (-24.9916, -17.3859) (-25.015, -17.422) (-25.0382, -17.4582) (-25.0613, -17.4946) (-25.0843, -17.5311) (-25.1072, -17.5677) (-25.13, -17.6044) (-25.1527, -17.6412) (-25.1753, -17.6781) (-25.1978, -17.7152) (-25.2201, -17.7523) (-25.2424, -17.7896) (-25.2645, -17.827) (-25.2821, -17.857) (-25.2953, -17.8795) (-25.304, -17.8946) (-25.3084, -17.9021) knots 0 0 0 0 0 0 0.01428571 0.02857143 0.04285714 0.05714286 0.07142857 0.08571429 0.1 0.11428571 0.12857143 0.14285714 0.15714286 0.17142857 0.18571429 0.2 0.21428571 0.22857143 0.24285714 0.25714286 0.27142857 0.28571429 0.3 0.31428571 0.32857143 0.34285714 0.35714286 0.37142857 0.38571429 0.4 0.41428571 0.42857143 0.44285714 0.45714286 0.47142857 0.48571429 0.5 0.51428571 0.52857143 0.54285714 0.55714286 0.57142857 0.58571429 0.6 0.61428571 0.62857143 0.64285714 0.65714286 0.67142857 0.68571429 0.7 0.71428571 0.72857143 0.74285714 0.75714286 0.77142857 0.78571429 0.8 0.81428571 0.82857143 0.84285714 0.85714286 0.87142857 0.88571429 0.9 0.91428571 0.92857143 0.94285714 0.95714286 0.97142857 0.98571429 1 1 1 1 1 1
  arc A6 (-25.3084, -17.9021) -> (-24.8466, -18.5377) centre (0, 0) ccw
  spline S13 degree 5 poles (-24.8466, -18.5377) (-24.8381, -18.5358) (-24.8211, -18.5322) (-24.7956, -18.5266) (-24.7616, -18.5191) (-24.7192, -18.5096) (-24.6769, -18.5) (-24.6347, -18.4902) (-24.5925, -18.4803) (-24.5504, -18.4702) (-24.5083, -18.46) (-24.4664, -18.4497) (-24.4245, -18.4392) (-24.3827, -18.4286) (-24.341, -18.4179) (-24.2994, -18.407) (-24.2578, -18.3959) (-24.2163, -18.3847) (-24.1749, -18.3734) (-24.1336, -18.3619) (-24.0924, -18.3503) (-24.0512, -18.3385) (-24.0101, -18.3265) (-23.9692, -18.3145) (-23.9283, -18.3022) (-23.8874, -18.2899) (-23.8467, -18.2773) (-23.8061, -18.2646) (-23.7656, -18.2518) (-23.7251, -18.2388) (-23.6848, -18.2256) (-23.6445, -18.2123) (-23.6044, -18.1988) (-23.5643, -18.1851) (-23.5243, -18.1713) (-23.4845, -18.1574) (-23.4447, -18.1432) (-23.405, -18.1289) (-23.3655, -18.1144) (-23.3261, -18.0998) (-23.2867, -18.0849) (-23.2475, -18.0699) (-23.2084, -18.0547) (-23.1694, -18.0394) (-23.1305, -18.0238) (-23.0917, -18.0081) (-23.0531, -17.9922) (-23.0146, -17.976) (-22.9762, -17.9597) (-22.938, -17.9432) (-22.8998, -17.9265) (-22.8618, -17.9096) (-22.824, -17.8925) (-22.7863, -17.8752) (-22.7487, -17.8576) (-22.7113, -17.8398) (-22.674, -17.8218) (-22.6369, -17.8036) (-22.6, -17.7851) (-22.5633, -17.7663) (-22.5267, -17.7473) (-22.4903, -17.7281) (-22.4541, -17.7086) (-22.4181, -17.6888) (-22.3823, -17.6687) (-22.3467, -17.6483) (-22.3114, -17.6275) (-22.2764, -17.6063) (-22.2418, -17.5846) (-22.2075, -17.5625) (-22.1736, -17.5398) (-22.1468, -17.5213) (-22.1268, -17.5072) (-22.1136, -17.4977) (-22.107, -17.4929) knots -1 -1 -1 -1 -1 -1 -0.98571429 -0.97142857 -0.95714286 -0.94285714 -0.92857143 -0.91428571 -0.9 -0.88571429 -0.87142857 -0.85714286 -0.84285714 -0.82857143 -0.81428571 -0.8 -0.78571429 -0.77142857 -0.75714286 -0.74285714 -0.72857143 -0.71428571 -0.7 -0.68571429 -0.67142857 -0.65714286 -0.64285714 -0.62857143 -0.61428571 -0.6 -0.58571429 -0.57142857 -0.55714286 -0.54285714 -0.52857143 -0.51428571 -0.5 -0.48571429 -0.47142857 -0.45714286 -0.44285714 -0.42857143 -0.41428571 -0.4 -0.38571429 -0.37142857 -0.35714286 -0.34285714 -0.32857143 -0.31428571 -0.3 -0.28571429 -0.27142857 -0.25714286 -0.24285714 -0.22857143 -0.21428571 -0.2 -0.18571429 -0.17142857 -0.15714286 -0.14285714 -0.12857143 -0.11428571 -0.1 -0.08571429 -0.07142857 -0.05714286 -0.04285714 -0.02857143 -0.01428571 0 0 0 0 0 0
  spline S14 degree 5 poles (-21.7069, -17.9869) (-21.713, -17.9924) (-21.725, -18.0033) (-21.743, -18.0199) (-21.7667, -18.0423) (-21.7959, -18.0708) (-21.8247, -18.0997) (-21.8531, -18.1291) (-21.8811, -18.1589) (-21.9088, -18.1891) (-21.9362, -18.2196) (-21.9632, -18.2505) (-21.9901, -18.2816) (-22.0167, -18.313) (-22.0431, -18.3446) (-22.0693, -18.3764) (-22.0952, -18.4084) (-22.121, -18.4407) (-22.1466, -18.4732) (-22.1719, -18.5059) (-22.1971, -18.5388) (-22.2221, -18.5719) (-22.2469, -18.6052) (-22.2715, -18.6386) (-22.2959, -18.6723) (-22.3202, -18.7061) (-22.3443, -18.7401) (-22.3682, -18.7742) (-22.392, -18.8086) (-22.4156, -18.843) (-22.4391, -18.8777) (-22.4624, -18.9125) (-22.4855, -18.9474) (-22.5085, -18.9825) (-22.5313, -19.0178) (-22.554, -19.0532) (-22.5765, -19.0887) (-22.5989, -19.1244) (-22.6212, -19.1602) (-22.6433, -19.1961) (-22.6652, -19.2322) (-22.687, -19.2684) (-22.7087, -19.3048) (-22.7303, -19.3413) (-22.7517, -19.3779) (-22.7729, -19.4146) (-22.7941, -19.4515) (-22.8151, -19.4885) (-22.8359, -19.5256) (-22.8567, -19.5628) (-22.8773, -19.6001) (-22.8977, -19.6376) (-22.9181, -19.6752) (-22.9383, -19.7128) (-22.9583, -19.7506) (-22.9783, -19.7886) (-22.9981, -19.8266) (-23.0178, -19.8647) (-23.0374, -19.903) (-23.0568, -19.9413) (-23.0762, -19.9798) (-23.0954, -20.0184) (-23.1144, -20.0571) (-23.1334, -20.0958) (-23.1522, -20.1347) (-23.1709, -20.1737) (-23.1895, -20.2128) (-23.208, -20.252) (-23.2263, -20.2913) (-23.2446, -20.3307) (-23.2627, -20.3702) (-23.2771, -20.4018) (-23.2878, -20.4256) (-23.2949, -20.4415) (-23.2985, -20.4495) knots 0 0 0 0 0 0 0.01428571 0.02857143 0.04285714 0.05714286 0.07142857 0.08571429 0.1 0.11428571 0.12857143 0.14285714 0.15714286 0.17142857 0.18571429 0.2 0.21428571 0.22857143 0.24285714 0.25714286 0.27142857 0.28571429 0.3 0.31428571 0.32857143 0.34285714 0.35714286 0.37142857 0.38571429 0.4 0.41428571 0.42857143 0.44285714 0.45714286 0.47142857 0.48571429 0.5 0.51428571 0.52857143 0.54285714 0.55714286 0.57142857 0.58571429 0.6 0.61428571 0.62857143 0.64285714 0.65714286 0.67142857 0.68571429 0.7 0.71428571 0.72857143 0.74285714 0.75714286 0.77142857 0.78571429 0.8 0.81428571 0.82857143 0.84285714 0.85714286 0.87142857 0.88571429 0.9 0.91428571 0.92857143 0.94285714 0.95714286 0.97142857 0.98571429 1 1 1 1 1 1
  arc A7 (-23.2985, -20.4495) -> (-22.7728, -21.0333) centre (0, 0) ccw
  spline S15 degree 5 poles (-22.7728, -21.0333) (-22.7645, -21.0306) (-22.748, -21.0252) (-22.7232, -21.017) (-22.6902, -21.006) (-22.649, -20.9921) (-22.6079, -20.9781) (-22.5669, -20.9639) (-22.526, -20.9497) (-22.4852, -20.9353) (-22.4445, -20.9207) (-22.4038, -20.9061) (-22.3633, -20.8913) (-22.3228, -20.8763) (-22.2825, -20.8613) (-22.2422, -20.8461) (-22.202, -20.8308) (-22.1619, -20.8153) (-22.1219, -20.7997) (-22.082, -20.7839) (-22.0423, -20.7681) (-22.0026, -20.7521) (-21.963, -20.7359) (-21.9235, -20.7196) (-21.8841, -20.7032) (-21.8448, -20.6866) (-21.8056, -20.6699) (-21.7665, -20.653) (-21.7275, -20.636) (-21.6887, -20.6188) (-21.6499, -20.6015) (-21.6113, -20.584) (-21.5728, -20.5664) (-21.5343, -20.5487) (-21.496, -20.5308) (-21.4579, -20.5127) (-21.4198, -20.4945) (-21.3818, -20.4761) (-21.344, -20.4575) (-21.3063, -20.4388) (-21.2688, -20.42) (-21.2313, -20.401) (-21.194, -20.3818) (-21.1568, -20.3624) (-21.1198, -20.3429) (-21.0829, -20.3232) (-21.0461, -20.3033) (-21.0095, -20.2833) (-20.973, -20.263) (-20.9367, -20.2426) (-20.9006, -20.222) (-20.8645, -20.2012) (-20.8287, -20.1802) (-20.793, -20.159) (-20.7575, -20.1377) (-20.7221, -20.1161) (-20.6869, -20.0943) (-20.652, -20.0722) (-20.6172, -20.05) (-20.5826, -20.0275) (-20.5482, -20.0048) (-20.514, -19.9818) (-20.48, -19.9587) (-20.4463, -19.9352) (-20.4128, -19.9115) (-20.3795, -19.8875) (-20.3466, -19.8631) (-20.314, -19.8384) (-20.2818, -19.8132) (-20.2501, -19.7876) (-20.2187, -19.7615) (-20.194, -19.7403) (-20.1756, -19.7242) (-20.1634, -19.7133) (-20.1574, -19.7079) knots -1 -1 -1 -1 -1 -1 -0.98571429 -0.97142857 -0.95714286 -0.94285714 -0.92857143 -0.91428571 -0.9 -0.88571429 -0.87142857 -0.85714286 -0.84285714 -0.82857143 -0.81428571 -0.8 -0.78571429 -0.77142857 -0.75714286 -0.74285714 -0.72857143 -0.71428571 -0.7 -0.68571429 -0.67142857 -0.65714286 -0.64285714 -0.62857143 -0.61428571 -0.6 -0.58571429 -0.57142857 -0.55714286 -0.54285714 -0.52857143 -0.51428571 -0.5 -0.48571429 -0.47142857 -0.45714286 -0.44285714 -0.42857143 -0.41428571 -0.4 -0.38571429 -0.37142857 -0.35714286 -0.34285714 -0.32857143 -0.31428571 -0.3 -0.28571429 -0.27142857 -0.25714286 -0.24285714 -0.22857143 -0.21428571 -0.2 -0.18571429 -0.17142857 -0.15714286 -0.14285714 -0.12857143 -0.11428571 -0.1 -0.08571429 -0.07142857 -0.05714286 -0.04285714 -0.02857143 -0.01428571 0 0 0 0 0 0
  spline S16 degree 5 poles (-19.7079, -20.1574) (-19.7133, -20.1634) (-19.7242, -20.1756) (-19.7403, -20.194) (-19.7615, -20.2187) (-19.7876, -20.2501) (-19.8132, -20.2818) (-19.8384, -20.314) (-19.8631, -20.3466) (-19.8875, -20.3795) (-19.9115, -20.4128) (-19.9352, -20.4463) (-19.9587, -20.48) (-19.9818, -20.514) (-20.0048, -20.5482) (-20.0275, -20.5826) (-20.05, -20.6172) (-20.0722, -20.652) (-20.0943, -20.6869) (-20.1161, -20.7221) (-20.1377, -20.7575) (-20.159, -20.793) (-20.1802, -20.8287) (-20.2012, -20.8645) (-20.222, -20.9006) (-20.2426, -20.9367) (-20.263, -20.973) (-20.2833, -21.0095) (-20.3033, -21.0461) (-20.3232, -21.0829) (-20.3429, -21.1198) (-20.3624, -21.1568) (-20.3818, -21.194) (-20.401, -21.2313) (-20.42, -21.2688) (-20.4388, -21.3063) (-20.4575, -21.344) (-20.4761, -21.3818) (-20.4945, -21.4198) (-20.5127, -21.4579) (-20.5308, -21.496) (-20.5487, -21.5343) (-20.5664, -21.5728) (-20.584, -21.6113) (-20.6015, -21.6499) (-20.6188, -21.6887) (-20.636, -21.7275) (-20.653, -21.7665) (-20.6699, -21.8056) (-20.6866, -21.8448) (-20.7032, -21.8841) (-20.7196, -21.9235) (-20.7359, -21.963) (-20.7521, -22.0026) (-20.7681, -22.0423) (-20.7839, -22.082) (-20.7997, -22.1219) (-20.8153, -22.1619) (-20.8308, -22.202) (-20.8461, -22.2422) (-20.8613, -22.2825) (-20.8763, -22.3228) (-20.8913, -22.3633) (-20.9061, -22.4038) (-20.9207, -22.4445) (-20.9353, -22.4852) (-20.9497, -22.526) (-20.9639, -22.5669) (-20.9781, -22.6079) (-20.9921, -22.649) (-21.006, -22.6902) (-21.017, -22.7232) (-21.0252, -22.748) (-21.0306, -22.7645) (-21.0333, -22.7728) knots 0 0 0 0 0 0 0.01428571 0.02857143 0.04285714 0.05714286 0.07142857 0.08571429 0.1 0.11428571 0.12857143 0.14285714 0.15714286 0.17142857 0.18571429 0.2 0.21428571 0.22857143 0.24285714 0.25714286 0.27142857 0.28571429 0.3 0.31428571 0.32857143 0.34285714 0.35714286 0.37142857 0.38571429 0.4 0.41428571 0.42857143 0.44285714 0.45714286 0.47142857 0.48571429 0.5 0.51428571 0.52857143 0.54285714 0.55714286 0.57142857 0.58571429 0.6 0.61428571 0.62857143 0.64285714 0.65714286 0.67142857 0.68571429 0.7 0.71428571 0.72857143 0.74285714 0.75714286 0.77142857 0.78571429 0.8 0.81428571 0.82857143 0.84285714 0.85714286 0.87142857 0.88571429 0.9 0.91428571 0.92857143 0.94285714 0.95714286 0.97142857 0.98571429 1 1 1 1 1 1
  arc A8 (-21.0333, -22.7728) -> (-20.4495, -23.2985) centre (0, 0) ccw
  spline S17 degree 5 poles (-20.4495, -23.2985) (-20.4415, -23.2949) (-20.4256, -23.2878) (-20.4018, -23.2771) (-20.3702, -23.2627) (-20.3307, -23.2446) (-20.2913, -23.2263) (-20.252, -23.208) (-20.2128, -23.1895) (-20.1737, -23.1709) (-20.1347, -23.1522) (-20.0958, -23.1334) (-20.0571, -23.1144) (-20.0184, -23.0954) (-19.9798, -23.0762) (-19.9413, -23.0568) (-19.903, -23.0374) (-19.8647, -23.0178) (-19.8266, -22.9981) (-19.7886, -22.9783) (-19.7506, -22.9583) (-19.7128, -22.9383) (-19.6752, -22.9181) (-19.6376, -22.8977) (-19.6001, -22.8773) (-19.5628, -22.8567) (-19.5256, -22.8359) (-19.4885, -22.8151) (-19.4515, -22.7941) (-19.4146, -22.7729) (-19.3779, -22.7517) (-19.3413, -22.7303) (-19.3048, -22.7087) (-19.2684, -22.687) (-19.2322, -22.6652) (-19.1961, -22.6433) (-19.1602, -22.6212) (-19.1244, -22.5989) (-19.0887, -22.5765) (-19.0532, -22.554) (-19.0178, -22.5313) (-18.9825, -22.5085) (-18.9474, -22.4855) (-18.9125, -22.4624) (-18.8777, -22.4391) (-18.843, -22.4156) (-18.8086, -22.392) (-18.7742, -22.3682) (-18.7401, -22.3443) (-18.7061, -22.3202) (-18.6723, -22.2959) (-18.6386, -22.2715) (-18.6052, -22.2469) (-18.5719, -22.2221) (-18.5388, -22.1971) (-18.5059, -22.1719) (-18.4732, -22.1466) (-18.4407, -22.121) (-18.4084, -22.0952) (-18.3764, -22.0693) (-18.3446, -22.0431) (-18.313, -22.0167) (-18.2816, -21.9901) (-18.2505, -21.9632) (-18.2196, -21.9362) (-18.1891, -21.9088) (-18.1589, -21.8811) (-18.1291, -21.8531) (-18.0997, -21.8247) (-18.0708, -21.7959) (-18.0423, -21.7667) (-18.0199, -21.743) (-18.0033, -21.725) (-17.9924, -21.713) (-17.9869, -21.7069) knots -1 -1 -1 -1 -1 -1 -0.98571429 -0.97142857 -0.95714286 -0.94285714 -0.92857143 -0.91428571 -0.9 -0.88571429 -0.87142857 -0.85714286 -0.84285714 -0.82857143 -0.81428571 -0.8 -0.78571429 -0.77142857 -0.75714286 -0.74285714 -0.72857143 -0.71428571 -0.7 -0.68571429 -0.67142857 -0.65714286 -0.64285714 -0.62857143 -0.61428571 -0.6 -0.58571429 -0.57142857 -0.55714286 -0.54285714 -0.52857143 -0.51428571 -0.5 -0.48571429 -0.47142857 -0.45714286 -0.44285714 -0.42857143 -0.41428571 -0.4 -0.38571429 -0.37142857 -0.35714286 -0.34285714 -0.32857143 -0.31428571 -0.3 -0.28571429 -0.27142857 -0.25714286 -0.24285714 -0.22857143 -0.21428571 -0.2 -0.18571429 -0.17142857 -0.15714286 -0.14285714 -0.12857143 -0.11428571 -0.1 -0.08571429 -0.07142857 -0.05714286 -0.04285714 -0.02857143 -0.01428571 0 0 0 0 0 0
  spline S18 degree 5 poles (-17.4929, -22.107) (-17.4977, -22.1136) (-17.5072, -22.1268) (-17.5213, -22.1468) (-17.5398, -22.1736) (-17.5625, -22.2075) (-17.5846, -22.2418) (-17.6063, -22.2764) (-17.6275, -22.3114) (-17.6483, -22.3467) (-17.6687, -22.3823) (-17.6888, -22.4181) (-17.7086, -22.4541) (-17.7281, -22.4903) (-17.7473, -22.5267) (-17.7663, -22.5633) (-17.7851, -22.6) (-17.8036, -22.6369) (-17.8218, -22.674) (-17.8398, -22.7113) (-17.8576, -22.7487) (-17.8752, -22.7863) (-17.8925, -22.824) (-17.9096, -22.8618) (-17.9265, -22.8998) (-17.9432, -22.938) (-17.9597, -22.9762) (-17.976, -23.0146) (-17.9922, -23.0531) (-18.0081, -23.0917) (-18.0238, -23.1305) (-18.0394, -23.1694) (-18.0547, -23.2084) (-18.0699, -23.2475) (-18.0849, -23.2867) (-18.0998, -23.3261) (-18.1144, -23.3655) (-18.1289, -23.405) (-18.1432, -23.4447) (-18.1574, -23.4845) (-18.1713, -23.5243) (-18.1851, -23.5643) (-18.1988, -23.6044) (-18.2123, -23.6445) (-18.2256, -23.6848) (-18.2388, -23.7251) (-18.2518, -23.7656) (-18.2646, -23.8061) (-18.2773, -23.8467) (-18.2899, -23.8874) (-18.3022, -23.9283) (-18.3145, -23.9692) (-18.3265, -24.0101) (-18.3385, -24.0512) (-18.3503, -24.0924) (-18.3619, -24.1336) (-18.3734, -24.1749) (-18.3847, -24.2163) (-18.3959, -24.2578) (-18.407, -24.2994) (-18.4179, -24.341) (-18.4286, -24.3827) (-18.4392, -24.4245) (-18.4497, -24.4664) (-18.46, -24.5083) (-18.4702, -24.5504) (-18.4803, -24.5925) (-18.4902, -24.6347) (-18.5, -24.6769) (-18.5096, -24.7192) (-18.5191, -24.7616) (-18.5266, -24.7956) (-18.5322, -24.8211) (-18.5358, -24.8381) (-18.5377, -24.8466) knots 0 0 0 0 0 0 0.01428571 0.02857143 0.04285714 0.05714286 0.07142857 0.08571429 0.1 0.11428571 0.12857143 0.14285714 0.15714286 0.17142857 0.18571429 0.2 0.21428571 0.22857143 0.24285714 0.25714286 0.27142857 0.28571429 0.3 0.31428571 0.32857143 0.34285714 0.35714286 0.37142857 0.38571429 0.4 0.41428571 0.42857143 0.44285714 0.45714286 0.47142857 0.48571429 0.5 0.51428571 0.52857143 0.54285714 0.55714286 0.57142857 0.58571429 0.6 0.61428571 0.62857143 0.64285714 0.65714286 0.67142857 0.68571429 0.7 0.71428571 0.72857143 0.74285714 0.75714286 0.77142857 0.78571429 0.8 0.81428571 0.82857143 0.84285714 0.85714286 0.87142857 0.88571429 0.9 0.91428571 0.92857143 0.94285714 0.95714286 0.97142857 0.98571429 1 1 1 1 1 1
  arc A9 (-18.5377, -24.8466) -> (-17.9021, -25.3084) centre (0, 0) ccw
  spline S19 degree 5 poles (-17.9021, -25.3084) (-17.8946, -25.304) (-17.8795, -25.2953) (-17.857, -25.2821) (-17.827, -25.2645) (-17.7896, -25.2424) (-17.7523, -25.2201) (-17.7152, -25.1978) (-17.6781, -25.1753) (-17.6412, -25.1527) (-17.6044, -25.13) (-17.5677, -25.1072) (-17.5311, -25.0843) (-17.4946, -25.0613) (-17.4582, -25.0382) (-17.422, -25.015) (-17.3859, -24.9916) (-17.3499, -24.9682) (-17.314, -24.9446) (-17.2783, -24.9209) (-17.2426, -24.8971) (-17.2072, -24.8732) (-17.1718, -24.8491) (-17.1365, -24.825) (-17.1014, -24.8007) (-17.0664, -24.7763) (-17.0316, -24.7518) (-16.9969, -24.7272) (-16.9623, -24.7024) (-16.9278, -24.6776) (-16.8935, -24.6526) (-16.8594, -24.6275) (-16.8253, -24.6022) (-16.7915, -24.5769) (-16.7577, -24.5514) (-16.7241, -24.5258) (-16.6907, -24.5) (-16.6574, -24.4742) (-16.6242, -24.4482) (-16.5913, -24.422) (-16.5584, -24.3958) (-16.5258, -24.3694) (-16.4933, -24.3429) (-16.4609, -24.3162) (-16.4288, -24.2894) (-16.3967, -24.2625) (-16.3649, -24.2354) (-16.3333, -24.2081) (-16.3018, -24.1808) (-16.2705, -24.1532) (-16.2394, -24.1256) (-16.2085, -24.0977) (-16.1778, -24.0698) (-16.1473, -24.0416) (-16.117, -24.0133) (-16.0869, -23.9849) (-16.057, -23.9562) (-16.0274, -23.9274) (-15.998, -23.8984) (-15.9689, -23.8692) (-15.94, -23.8398) (-15.9113, -23.8103) (-15.8829, -23.7806) (-15.8547, -23.7506) (-15.8269, -23.7205) (-15.7993, -23.6901) (-15.7722, -23.6594) (-15.7455, -23.6284) (-15.7192, -23.5971) (-15.6935, -23.5654) (-15.6682, -23.5334) (-15.6485, -23.5075) (-15.6338, -23.4879) (-15.6242, -23.4747) (-15.6194, -23.4682) knots -1 -1 -1 -1 -1 -1 -0.98571429 -0.97142857 -0.95714286 -0.94285714 -0.92857143 -0.91428571 -0.9 -0.88571429 -0.87142857 -0.85714286 -0.84285714 -0.82857143 -0.81428571 -0.8 -0.78571429 -0.77142857 -0.75714286 -0.74285714 -0.72857143 -0.71428571 -0.7 -0.68571429 -0.67142857 -0.65714286 -0.64285714 -0.62857143 -0.61428571 -0.6 -0.58571429 -0.57142857 -0.55714286 -0.54285714 -0.52857143 -0.51428571 -0.5 -0.48571429 -0.47142857 -0.45714286 -0.44285714 -0.42857143 -0.41428571 -0.4 -0.38571429 -0.37142857 -0.35714286 -0.34285714 -0.32857143 -0.31428571 -0.3 -0.28571429 -0.27142857 -0.25714286 -0.24285714 -0.22857143 -0.21428571 -0.2 -0.18571429 -0.17142857 -0.15714286 -0.14285714 -0.12857143 -0.11428571 -0.1 -0.08571429 -0.07142857 -0.05714286 -0.04285714 -0.02857143 -0.01428571 0 0 0 0 0 0
  spline S20 degree 5 poles (-15.0862, -23.8144) (-15.0903, -23.8215) (-15.0984, -23.8356) (-15.1103, -23.8569) (-15.126, -23.8855) (-15.1449, -23.9216) (-15.1634, -23.958) (-15.1813, -23.9948) (-15.1988, -24.0318) (-15.2158, -24.069) (-15.2324, -24.1065) (-15.2486, -24.1442) (-15.2645, -24.1821) (-15.2801, -24.2202) (-15.2954, -24.2584) (-15.3105, -24.2968) (-15.3253, -24.3353) (-15.3398, -24.3739) (-15.3541, -24.4127) (-15.3681, -24.4516) (-15.3819, -24.4907) (-15.3954, -24.5299) (-15.4087, -24.5692) (-15.4218, -24.6087) (-15.4346, -24.6482) (-15.4473, -24.6879) (-15.4597, -24.7276) (-15.4719, -24.7675) (-15.4839, -24.8075) (-15.4957, -24.8476) (-15.5073, -24.8878) (-15.5187, -24.9281) (-15.5299, -24.9685) (-15.5409, -25.009) (-15.5517, -25.0495) (-15.5624, -25.0902) (-15.5728, -25.131) (-15.5831, -25.1718) (-15.5932, -25.2128) (-15.6031, -25.2538) (-15.6128, -25.2949) (-15.6224, -25.3361) (-15.6318, -25.3773) (-15.641, -25.4187) (-15.65, -25.4601) (-15.6589, -25.5016) (-15.6676, -25.5432) (-15.6762, -25.5849) (-15.6845, -25.6266) (-15.6927, -25.6684) (-15.7008, -25.7103) (-15.7087, -25.7522) (-15.7164, -25.7942) (-15.724, -25.8363) (-15.7314, -25.8785) (-15.7387, -25.9207) (-15.7458, -25.963) (-15.7527, -26.0054) (-15.7595, -26.0478) (-15.7661, -26.0903) (-15.7726, -26.1329) (-15.779, -26.1755) (-15.7852, -26.2181) (-15.7912, -26.2609) (-15.7971, -26.3037) (-15.8028, -26.3466) (-15.8084, -26.3895) (-15.8139, -26.4325) (-15.8192, -26.4755) (-15.8244, -26.5186) (-15.8294, -26.5617) (-15.8333, -26.5963) (-15.8361, -26.6223) (-15.838, -26.6396) (-15.8389, -26.6482) knots 0 0 0 0 0 0 0.01428571 0.02857143 0.04285714 0.05714286 0.07142857 0.08571429 0.1 0.11428571 0.12857143 0.14285714 0.15714286 0.17142857 0.18571429 0.2 0.21428571 0.22857143 0.24285714 0.25714286 0.27142857 0.28571429 0.3 0.31428571 0.32857143 0.34285714 0.35714286 0.37142857 0.38571429 0.4 0.41428571 0.42857143 0.44285714 0.45714286 0.47142857 0.48571429 0.5 0.51428571 0.52857143 0.54285714 0.55714286 0.57142857 0.58571429 0.6 0.61428571 0.62857143 0.64285714 0.65714286 0.67142857 0.68571429 0.7 0.71428571 0.72857143 0.74285714 0.75714286 0.77142857 0.78571429 0.8 0.81428571 0.82857143 0.84285714 0.85714286 0.87142857 0.88571429 0.9 0.91428571 0.92857143 0.94285714 0.95714286 0.97142857 0.98571429 1 1 1 1 1 1
  arc A10 (-15.8389, -26.6482) -> (-15.1586, -27.041) centre (0, 0) ccw